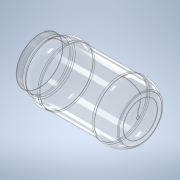
# Autodesk Inventor part: Container_2L
Saved by Autodesk Inventor 2020 (Build 240168000, 168)
## iProperties
Created: 2021-04-27
Part Number: Container_2L
Material: Polycarbonate, Clear
Document SubType Name: Modeling
Designer: Workshop
Density: 1.2 g/cm^3
Appearance: Polycarbonate - Clear
Author: Workshop
Autodesk Inventor part; units mm, degrees
ref_plane "YZ Plane" through (0, 0, 0) normal (1, 0, 0) x (0, 1, 0)
ref_plane "XZ Plane" through (0, 0, 0) normal (0, 1, 0) x (-1, 0, 0)
ref_plane "XY Plane" through (0, 0, 0) normal (0, 0, 1) x (1, 0, 0)
sketch "Sketch1" plane through (0, 0, 0) normal (0, 0, 1) x (1, 0, 0)
  line L0 (0, 0) -> (0, 48)
  line L1 (0, 48) -> (19, 48)
  line L2 (0, 0) -> (954, 0)
  line L3 (55, 56) -> (167.3, 56)
  line L4 (207.3, 0) -> (207.3, 45) construction
  line L5 (-18, 58.25) -> (230, 58.25) construction
  line L6 (19, 48) -> (34.3428, 62.1451) construction
  line L7 (34.3428, 62.1451) -> (49.3631, 58.25) construction
  line L8 (49.3631, 58.25) -> (55, 56) construction
  spline S0 degree 3 poles (19, 48) (34.3428, 62.1451) (49.3631, 58.25) (55, 56) knots 1 1 1 1 2 2 2 2
  line L9 (167.3, 56) -> (179.4553, 62.9349) construction
  line L10 (179.4553, 62.9349) -> (204.8001, 52.2901) construction
  line L11 (204.8001, 52.2901) -> (207.3, 45) construction
  spline S1 degree 3 poles (167.3, 56) (179.4553, 62.9349) (204.8001, 52.2901) (207.3, 45) knots 1 1 1 1 2 2 2 2
  line L12 (207.3, 45) -> (207.3, 35)
  line L13 (0, 0) -> (202.3, 0) construction
  line L14 (202.3, 0) -> (202.3, 3)
  line L15 (202.3, 3) -> (202.3, 13) construction
  line L16 (202.3, 13) -> (203, 17) construction
  line L17 (203, 17) -> (207.3, 20) construction
  line L18 (207.3, 20) -> (207.3, 35) construction
  spline S2 degree 4 poles (202.3, 3) (202.3, 13) (203, 17) (207.3, 20) (207.3, 35) knots 1 1 1 1 1 2 2 2 2 2
  line L19 (0, 0) -> (202.3, 0)
  dimension "d1" = 48
  dimension "d2" = 19
  dimension "d3" = 55
  dimension "d4" = 112
  dimension "d5" = 207.3
  dimension "d7" = 116.5
  dimension "d8" = 45
  dimension "d9" = 10
  dimension "d11" = 3
  dimension "d12" = 5
  dimension "d22" = 112.3
  constraints: 20 end point, 5 horizontal, 5 point on line, 3 vertical, 2 perpendicular, 1 collinear, 9 other
  measures "d1" distance of L0.start L0.end
  measures "d2" distance of L0.end L1.end
  measures "d3" distance from line of L0 L3.start
  measures "d4" diameter of L3 L2
  measures "d5" distance between parallel lines of L4 L0
  measures "d7" diameter of L5 L2
  measures "d8" distance of L4.start L4.end
  measures "d9" distance of L4.end L12.end
  measures "d11" distance of L13.end L14.end
  measures "d12" distance between parallel lines of L4 L14
  measures "d22" distance of L3.start L3.end
revolve "Revolution1" add sketch "Sketch1" angle 360 about axis through (0, 0, 0) along (1, 0, 0)
shell "Shell1" thickness 1 removed faces 1 at (0, 14.7854, 4.691)
fillet "Fillet1" radius 15 1 edges at (19, -48, 0)
fillet "Fillet2" radius 15 1 edges at (55, -56, 0)
fillet "Fillet3" radius 15 1 edges at (167.3, -56, 0)
fillet "Fillet4" radius 5 2 edges at (207.3, -45, 0) (207.3, -35, 0)
fillet "Fillet5" radius 5 1 edges at (19.3906, -47, 0.0003)
thread "Thread1" size "M100x6" class "6g" standard "ANSI Metric M Profile" full length
body "Solid1"
